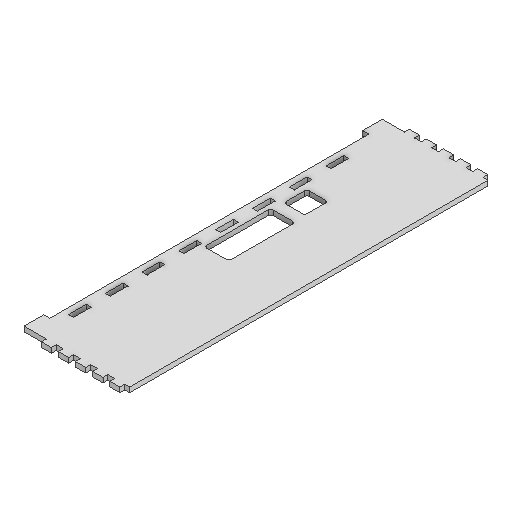
# Autodesk Inventor part: back
Saved by Autodesk Inventor 2025.2 (Build 292293000, 293)
## iProperties
Created: 2025-12-09
Part Number: back
Material: Generic
Document SubType Name: Modeling
Designer: hazem
Density: 1 g/cm^3
Appearance: Default
Author: hazem
Autodesk Inventor part; units mm, degrees
ref_plane "YZ Plane" through (0, 0, 0) normal (1, 0, 0) x (0, 1, 0)
ref_plane "XZ Plane" through (0, 0, 0) normal (0, 1, 0) x (-1, 0, 0)
ref_plane "XY Plane" through (0, 0, 0) normal (0, 0, 1) x (1, 0, 0)
sketch "Sketch1" plane through (0, 0, 0) normal (0, 1, 0) x (-1, 0, 0)
  line L0 (-71.6259, 7.6308) -> (8.4741, 7.6308)
  line L1 (8.4741, 7.6308) -> (8.4741, -292.3692)
  line L2 (8.4741, -292.3692) -> (-71.6259, -292.3692)
  line L3 (-71.6259, -292.3692) -> (-71.6259, 7.6308)
  point P0 (0, 0)
  constraints: 8 end point, 2 parallel, 1 horizontal, 1 perpendicular
extrude "Extrusion1" add sketch "Sketch1" along normal blind 4
sketch "Sketch2" plane through (0, 0, 0) normal (0, -1, 0) x (1, 0, 0)
  line L0 (-0.3741, 7.6308) -> (-18.4741, 7.6308) construction
  line L1 (-0.3741, 3.6308) -> (-0.3741, 7.6308) construction
  line L2 (7.6259, 7.6308) -> (7.6259, 3.6308) construction
  line L3 (13.6259, 3.6308) -> (7.6259, 3.6308) construction
  line L4 (13.6259, 3.6308) -> (13.6259, 7.6308) construction
  line L5 (21.6259, 7.6308) -> (21.6259, 3.6308) construction
  line L6 (27.6259, 3.6308) -> (21.6259, 3.6308) construction
  line L7 (27.6259, 3.6308) -> (27.6259, 7.6308) construction
  line L8 (35.6259, 7.6308) -> (35.6259, 3.6308) construction
  line L9 (41.6259, 3.6308) -> (35.6259, 3.6308) construction
  line L10 (41.6259, 3.6308) -> (41.6259, 7.6308) construction
  line L11 (49.6259, 7.6308) -> (49.6259, 3.6308) construction
  line L12 (55.6259, 3.6308) -> (49.6259, 3.6308) construction
  line L13 (55.6259, 3.6308) -> (55.6259, 7.6308) construction
  line L14 (63.6259, 7.6308) -> (63.6259, 3.6308) construction
  line L15 (67.6259, 3.6308) -> (63.6259, 3.6308) construction
  line L16 (67.6259, 7.6308) -> (67.6259, -292.3692) projected
  line L17 (71.6259, 7.6308) -> (71.6259, -292.3692) projected
  line L18 (67.6259, 7.6308) -> (67.6259, -292.3692) projected
  line L19 (71.6259, 7.6308) -> (71.6259, -292.3692) projected
  line L20 (67.6259, 7.6308) -> (67.6259, -292.3692) projected
  line L21 (71.6259, 7.6308) -> (71.6259, -292.3692) projected
  line L22 (67.6259, 7.6308) -> (67.6259, -292.3692) projected
  line L23 (71.6259, 7.6308) -> (71.6259, -292.3692) projected
  line L24 (67.6259, 7.6308) -> (67.6259, -292.3692) projected
  line L25 (71.6259, 7.6308) -> (71.6259, -292.3692) projected
  line L26 (67.6259, 7.6308) -> (67.6259, -292.3692) projected
  line L27 (71.6259, 7.6308) -> (71.6259, -292.3692) projected
  line L28 (67.6259, 7.6308) -> (67.6259, -292.3692) projected
  line L29 (71.6259, 7.6308) -> (71.6259, -292.3692) projected
  line L30 (67.6259, 7.6308) -> (67.6259, -292.3692) projected
  line L31 (71.6259, 7.6308) -> (71.6259, -292.3692) projected
  line L32 (67.6259, 7.6308) -> (67.6259, -292.3692) projected
  line L33 (71.6259, 7.6308) -> (71.6259, -292.3692) projected
  line L34 (67.6259, 7.6308) -> (67.6259, -292.3692) projected
  line L35 (71.6259, 7.6308) -> (71.6259, -292.3692) projected
  line L36 (13.5259, -288.3692) -> (7.5259, -288.3692) projected
  line L37 (55.5259, -292.3692) -> (55.5259, -288.3692) projected
  line L38 (55.5259, -288.3692) -> (49.5259, -288.3692) projected
  line L39 (49.5259, -288.3692) -> (49.5259, -292.3692) projected
  line L40 (41.5259, -288.3692) -> (35.5259, -288.3692) projected
  line L41 (41.5259, -292.3692) -> (41.5259, -288.3692) projected
  line L42 (35.5259, -288.3692) -> (35.5259, -292.3692) projected
  line L43 (27.5259, -288.3692) -> (21.5259, -288.3692) projected
  line L44 (27.5259, -292.3692) -> (27.5259, -288.3692) projected
  line L45 (21.5259, -288.3692) -> (21.5259, -292.3692) projected
  line L46 (13.5259, -288.3692) -> (7.5259, -288.3692) projected
  line L47 (13.5259, -292.3692) -> (13.5259, -288.3692) projected
  line L48 (7.5259, -288.3692) -> (7.5259, -292.3692) projected
  line L49 (-8.4741, -292.3692) -> (-8.4741, 7.6308) projected
  line L50 (-8.4741, -22.3692) -> (-8.4741, -37.3692) projected
  line L51 (-8.4741, -37.3692) -> (-4.4741, -37.3692) projected
  line L52 (-4.4741, -22.3692) -> (-4.4741, -37.3692) projected
  line L53 (-8.4741, -22.3692) -> (-4.4741, -22.3692) projected
  line L54 (-8.4741, -52.3692) -> (-8.4741, -67.3692) projected
  line L55 (-8.4741, -67.3692) -> (-4.4741, -67.3692) projected
  line L56 (-4.4741, -52.3692) -> (-4.4741, -67.3692) projected
  line L57 (-8.4741, -52.3692) -> (-4.4741, -52.3692) projected
  line L58 (-8.4741, -82.3692) -> (-8.4741, -97.3692) projected
  line L59 (-8.4741, -97.3692) -> (-4.4741, -97.3692) projected
  line L60 (-4.4741, -82.3692) -> (-4.4741, -97.3692) projected
  line L61 (-8.4741, -82.3692) -> (-4.4741, -82.3692) projected
  line L62 (-8.4741, -112.3692) -> (-8.4741, -127.3692) projected
  line L63 (-8.4741, -127.3692) -> (-4.4741, -127.3692) projected
  line L64 (-4.4741, -112.3692) -> (-4.4741, -127.3692) projected
  line L65 (-8.4741, -112.3692) -> (-4.4741, -112.3692) projected
  line L66 (-8.4741, -142.3692) -> (-8.4741, -157.3692) projected
  line L67 (-8.4741, -157.3692) -> (-4.4741, -157.3692) projected
  line L68 (-4.4741, -142.3692) -> (-4.4741, -157.3692) projected
  line L69 (-8.4741, -142.3692) -> (-4.4741, -142.3692) projected
  line L70 (-8.4741, -172.3692) -> (-8.4741, -187.3692) projected
  line L71 (-8.4741, -187.3692) -> (-4.4741, -187.3692) projected
  line L72 (-4.4741, -172.3692) -> (-4.4741, -187.3692) projected
  line L73 (-8.4741, -172.3692) -> (-4.4741, -172.3692) projected
  line L74 (-8.4741, -202.3692) -> (-8.4741, -217.3692) projected
  line L75 (-8.4741, -217.3692) -> (-4.4741, -217.3692) projected
  line L76 (-4.4741, -202.3692) -> (-4.4741, -217.3692) projected
  line L77 (-8.4741, -202.3692) -> (-4.4741, -202.3692) projected
  line L78 (-8.4741, -232.3692) -> (-8.4741, -247.3692) projected
  line L79 (-8.4741, -247.3692) -> (-4.4741, -247.3692) projected
  line L80 (-4.4741, -232.3692) -> (-4.4741, -247.3692) projected
  line L81 (-8.4741, -232.3692) -> (-4.4741, -232.3692) projected
  line L82 (71.6259, -37.1192) -> (67.6259, -37.1192)
  line L83 (67.6259, -22.6192) -> (71.6259, -22.6192)
  line L84 (67.6259, -52.6192) -> (71.6259, -52.6192)
  line L85 (71.6259, -67.1192) -> (67.6259, -67.1192)
  line L86 (67.6259, -82.6192) -> (71.6259, -82.6192)
  line L87 (71.6259, -97.1192) -> (67.6259, -97.1192)
  line L88 (67.6259, -112.6192) -> (71.6259, -112.6192)
  line L89 (71.6259, -127.1192) -> (67.6259, -127.1192)
  line L90 (67.6259, -142.6192) -> (71.6259, -142.6192)
  line L91 (71.6259, -157.1192) -> (67.6259, -157.1192)
  line L92 (67.6259, -172.6192) -> (71.6259, -172.6192)
  line L93 (71.6259, -187.1192) -> (67.6259, -187.1192)
  line L94 (67.6259, -202.6192) -> (71.6259, -202.6192)
  line L95 (71.6259, -217.1192) -> (67.6259, -217.1192)
  line L96 (67.6259, -232.6192) -> (71.6259, -232.6192)
  line L97 (71.6259, -247.1192) -> (67.6259, -247.1192)
  line L98 (67.6259, -262.6192) -> (71.6259, -262.6192)
  line L99 (71.6259, -277.1192) -> (67.6259, -277.1192)
  line L100 (-4.4741, -22.6192) -> (-8.4741, -22.6192)
  line L101 (-4.4741, -37.1192) -> (-8.4741, -37.1192)
  line L102 (-4.4741, -52.6192) -> (-8.4741, -52.6192)
  line L103 (-4.4741, -67.1192) -> (-8.4741, -67.1192)
  line L104 (-4.4741, -82.6192) -> (-8.4741, -82.6192)
  line L105 (-4.4741, -97.1192) -> (-8.4741, -97.1192)
  line L106 (-4.4741, -112.6192) -> (-8.4741, -112.6192)
  line L107 (-4.4741, -127.1192) -> (-8.4741, -127.1192)
  line L108 (-4.4741, -142.6192) -> (-8.4741, -142.6192)
  line L109 (-4.4741, -157.1192) -> (-8.4741, -157.1192)
  line L110 (-4.4741, -172.6192) -> (-8.4741, -172.6192)
  line L111 (-4.4741, -187.1192) -> (-8.4741, -187.1192)
  line L112 (-4.4741, -202.6192) -> (-8.4741, -202.6192)
  line L113 (-4.4741, -217.1192) -> (-8.4741, -217.1192)
  line L114 (-4.4741, -232.6192) -> (-8.4741, -232.6192)
  line L115 (-4.4741, -247.1192) -> (-8.4741, -247.1192)
  line L116 (7.8759, 7.6308) -> (7.8759, 3.6308)
  line L117 (13.3759, 3.6308) -> (13.3759, 7.6308)
  line L118 (21.8759, 7.6308) -> (21.8759, 3.6308)
  line L119 (27.3759, 3.6308) -> (27.3759, 7.6308)
  line L120 (35.8759, 7.6308) -> (35.8759, 3.6308)
  line L121 (41.3759, 3.6308) -> (41.3759, 7.6308)
  line L122 (49.8759, 7.6308) -> (49.8759, 3.6308)
  line L123 (55.3759, 3.6308) -> (55.3759, 7.6308)
  line L124 (7.7759, -292.3692) -> (7.7759, -288.3692)
  line L125 (13.2759, -288.3692) -> (13.2759, -292.3692)
  line L126 (21.7759, -292.3692) -> (21.7759, -288.3692)
  line L127 (27.2759, -288.3692) -> (27.2759, -292.3692)
  line L128 (35.7759, -292.3692) -> (35.7759, -288.3692)
  line L129 (41.2759, -288.3692) -> (41.2759, -292.3692)
  line L130 (49.7759, -292.3692) -> (49.7759, -288.3692)
  line L131 (55.2759, -288.3692) -> (55.2759, -292.3692)
  line L132 (13.6259, 3.6308) -> (7.6259, 3.6308) projected
  line L133 (27.6259, 3.6308) -> (21.6259, 3.6308) projected
  line L134 (41.6259, 3.6308) -> (35.6259, 3.6308) projected
  line L135 (55.6259, 3.6308) -> (49.6259, 3.6308) projected
  line L136 (71.6259, -292.3692) -> (-8.4741, -292.3692) projected
  line L137 (-0.3741, 3.6308) -> (-0.3741, 7.6308) projected
  line L138 (-8.4741, 7.6308) -> (71.6259, 7.6308) projected
  line L139 (71.6259, 7.6308) -> (71.6259, -292.3692) projected
  line L140 (63.6259, 7.6308) -> (63.6259, 3.6308) projected
  line L141 (67.6259, 3.6308) -> (63.6259, 3.6308) projected
  line L142 (-0.3741, 3.6308) -> (-18.4741, 3.6308) projected
  line L143 (-18.4741, 7.6308) -> (-18.4741, 3.6308) projected
  line L144 (-0.3741, 7.6308) -> (-18.4741, 7.6308) projected
  line L145 (-0.3741, 3.6308) -> (-0.3741, 7.6308) projected
  line L146 (-0.3741, 7.6308) -> (-18.4741, 7.6308) projected
  line L147 (-18.4741, 7.6308) -> (-18.4741, 3.6308) projected
  line L148 (-0.3741, 3.6308) -> (-18.4741, 3.6308) projected
  line L149 (-0.4741, -292.3692) -> (-0.4741, -288.3692) projected
  line L150 (-0.4741, -288.3692) -> (-18.4741, -288.3692) projected
  line L151 (-18.4741, -292.3692) -> (-18.4741, -288.3692) projected
  line L152 (-0.4741, -292.3692) -> (-18.4741, -292.3692) projected
  line L153 (15.6627, -189.1692) -> (2.2391, -189.1692)
  line L154 (0.3759, -191.0324) -> (0.3759, -206.206)
  line L155 (2.2391, -208.0692) -> (15.6627, -208.0692)
  line L156 (17.5259, -206.206) -> (17.5259, -191.0324)
  arc A0 (17.5259, -191.0324) -> (15.6627, -189.1692) centre (15.6627, -191.0324) ccw
  arc A1 (2.2391, -189.1692) -> (0.3759, -191.0324) centre (2.2391, -191.0324) ccw
  arc A2 (15.6627, -208.0692) -> (17.5259, -206.206) centre (15.6627, -206.206) ccw
  arc A3 (0.3759, -206.206) -> (2.2391, -208.0692) centre (2.2391, -206.206) ccw
  line L157 (16.9509, -125.8692) -> (0.9509, -125.8692)
  line L158 (-1.0491, -127.8692) -> (-1.0491, -177.8692)
  line L159 (0.9509, -179.8692) -> (16.9509, -179.8692)
  line L160 (18.9509, -177.8692) -> (18.9509, -127.8692)
  arc A4 (18.9509, -127.8692) -> (16.9509, -125.8692) centre (16.9509, -127.8692) ccw
  arc A5 (0.9509, -125.8692) -> (-1.0491, -127.8692) centre (0.9509, -127.8692) ccw
  arc A6 (16.9509, -179.8692) -> (18.9509, -177.8692) centre (16.9509, -177.8692) ccw
  arc A7 (-1.0491, -177.8692) -> (0.9509, -179.8692) centre (0.9509, -177.8692) ccw
  line L161 (67.6259, -292.3692) -> (71.6259, -292.3692) projected
  line L162 (67.6259, 7.6308) -> (71.6259, 7.6308) projected
  line L163 (67.6259, -292.3692) -> (71.6259, -292.3692) projected
  line L164 (67.6259, 7.6308) -> (71.6259, 7.6308) projected
  line L165 (67.6259, -292.3692) -> (71.6259, -292.3692) projected
  line L166 (67.6259, 7.6308) -> (71.6259, 7.6308) projected
  line L167 (67.6259, -292.3692) -> (71.6259, -292.3692) projected
  line L168 (67.6259, 7.6308) -> (71.6259, 7.6308) projected
  line L169 (67.6259, -292.3692) -> (71.6259, -292.3692) projected
  line L170 (67.6259, 7.6308) -> (71.6259, 7.6308) projected
  line L171 (67.6259, -292.3692) -> (71.6259, -292.3692) projected
  line L172 (67.6259, 7.6308) -> (71.6259, 7.6308) projected
  line L173 (67.6259, -292.3692) -> (71.6259, -292.3692) projected
  line L174 (67.6259, 7.6308) -> (71.6259, 7.6308) projected
  line L175 (67.6259, -292.3692) -> (71.6259, -292.3692) projected
  line L176 (67.6259, 7.6308) -> (71.6259, 7.6308) projected
  line L177 (67.6259, -292.3692) -> (71.6259, -292.3692) projected
  line L178 (67.6259, 7.6308) -> (71.6259, 7.6308) projected
  line L179 (67.6259, -292.3692) -> (71.6259, -292.3692) projected
  line L180 (67.6259, 7.6308) -> (71.6259, 7.6308) projected
  point P0 (0, 0)
  point P1 (71.6259, -7.3692)
  point P2 (71.6259, -37.3692)
  point P3 (71.6259, -22.3692)
  point P4 (71.6259, -67.3692)
  point P5 (71.6259, -52.3692)
  point P6 (71.6259, -97.3692)
  point P7 (71.6259, -82.3692)
  point P8 (71.6259, -127.3692)
  point P9 (71.6259, -112.3692)
  point P10 (71.6259, -157.3692)
  point P11 (71.6259, -142.3692)
  point P12 (71.6259, -187.3692)
  point P13 (71.6259, -172.3692)
  point P14 (71.6259, -217.3692)
  point P15 (71.6259, -202.3692)
  point P16 (71.6259, -247.3692)
  point P17 (71.6259, -232.3692)
  point P18 (71.6259, -277.3692)
  point P19 (71.6259, -262.3692)
  point P20 (67.6259, -97.1192)
  point P21 (71.6259, -97.1192)
  point P22 (71.6259, -82.6192)
  point P23 (67.6259, -82.6192)
  point P24 (67.6259, -127.1192)
  point P25 (71.6259, -127.1192)
  point P26 (71.6259, -112.6192)
  point P27 (67.6259, -112.6192)
  point P28 (67.6259, -157.1192)
  point P29 (71.6259, -157.1192)
  point P30 (71.6259, -142.6192)
  point P31 (67.6259, -142.6192)
  point P32 (67.6259, -187.1192)
  point P33 (71.6259, -187.1192)
  point P34 (71.6259, -172.6192)
  point P35 (67.6259, -172.6192)
  point P36 (67.6259, -217.1192)
  point P37 (71.6259, -217.1192)
  point P38 (71.6259, -202.6192)
  point P39 (67.6259, -202.6192)
  point P40 (67.6259, -247.1192)
  point P41 (71.6259, -247.1192)
  point P42 (71.6259, -232.6192)
  point P43 (67.6259, -232.6192)
  point P44 (67.6259, -277.1192)
  point P45 (71.6259, -277.1192)
  point P46 (71.6259, -262.6192)
  point P47 (67.6259, -262.6192)
  point P48 (-8.4741, -247.1192)
  point P49 (-4.4741, -247.1192)
  point P50 (-4.4741, -232.6192)
  point P51 (-8.4741, -232.6192)
  point P52 (-8.4741, -217.1192)
  point P53 (-4.4741, -217.1192)
  point P54 (-4.4741, -202.6192)
  point P55 (-8.4741, -202.6192)
  point P56 (-8.4741, -187.1192)
  point P57 (-4.4741, -187.1192)
  point P58 (-4.4741, -172.6192)
  point P59 (-8.4741, -172.6192)
  point P60 (-8.4741, -157.1192)
  point P61 (-4.4741, -157.1192)
  point P62 (-4.4741, -142.6192)
  point P63 (-8.4741, -142.6192)
  point P64 (-8.4741, -127.1192)
  point P65 (-4.4741, -127.1192)
  point P66 (-4.4741, -112.6192)
  point P67 (-8.4741, -112.6192)
  point P68 (-8.4741, -97.1192)
  point P69 (-4.4741, -97.1192)
  point P70 (-4.4741, -82.6192)
  point P71 (-8.4741, -82.6192)
  point P72 (-8.4741, -67.1192)
  point P73 (-4.4741, -67.1192)
  point P74 (-4.4741, -52.6192)
  point P75 (-8.4741, -52.6192)
  point P76 (-8.4741, -37.1192)
  point P77 (-8.4741, -22.6192)
  point P78 (67.6259, -67.1192)
  point P79 (71.6259, -67.1192)
  point P80 (71.6259, -52.6192)
  point P81 (67.6259, -52.6192)
  point P82 (8.9509, -189.1692)
  point P83 (8.9509, -179.8692)
  point P84 (67.6259, -292.3692)
  point P85 (67.6259, 3.6308)
  point P86 (67.6259, 7.6308)
  point P87 (71.6259, 3.6308)
  point P88 (67.6259, -288.3692)
  point P89 (71.6259, -288.3692)
  point P90 (-8.4741, 3.6308)
  point P91 (21.7759, -288.3692)
  point P92 (35.7759, -288.3692)
  point P93 (49.7759, -288.3692)
  point P94 (-8.4741, -288.3692)
  dimension "d7" = 30
  dimension "d15" = 30
  dimension "d20" = 0.25
  dimension "d23" = 14
  dimension "d28" = 0.25
  dimension "d31" = 14
  dimension "d49" = 2
  dimension "d50" = 50
  dimension "d51" = 20
  constraints: 118 end point, 16 point on circle, 16 tangent, 12 point on line, 8 centre point, 6 equal radius, 4 horizontal, 4 parallel, 4 perpendicular, 2 collinear, 2 midpoint, 2 vertical, 1 vertical alignment, 130 other
  measures "d7" distance of L83.start L84.start
  measures "d15" distance of L100.start L102.start
  measures "d20" distance between parallel lines of L2 L116
  measures "d23" distance of L116.start L118.start
  measures "d28" distance between parallel lines of L48 L124
  measures "d31" distance of L124.start L126.start
  measures "d49" radius of A4
  measures "d50" distance of L160.start L160.end
  measures "d51" distance between parallel lines of L158 L160
extrude "Extrusion2" cut sketch "Sketch2" against normal through all contours L138 L17 L83 L16 | L16 L141 L140 L138 | L83 L17 L82 L16 | L123 L135 L122 L138 | L82 L17 L84 L16 | L84 L17 L85 L16 | L121 L134 L120 L138 | L85 L17 L86 L16 | L86 L17 L87 L16 | L119 L133 L118 L138 | L87 L17 L88 L16 | L88 L17 L89 L16 | L117 L132 L116 L138 | L89 L17 L90 L16 | L90 L17 L91 L16 | L137 L142 L49 L138 | L91 L17 L92 L16 | L92 L17 L93 L16 | L93 L17 L94 L16 | L94 L17 L95 L16 | L100 L52 L101 L49 | L95 L17 L96 L16 | L96 L17 L97 L16 | L97 L17 L98 L16 | L98 L17 L99 L16 | L102 L56 L103 L49 | L99 L17 L136 L16 | L136 L130 L38 L131 | L104 L60 L105 L49 | L136 L128 L40 L129 | L106 L64 L107 L49 | L136 L126 L43 L127 | L108 L68 L109 L49 | L136 L124 L36 L125 | L110 L72 L111 L49 | L136 L49 L150 L149 | L112 L76 L113 L49 | L49 L114 L80 L115 | A0 L156 A2 L155 A3 L154 A1 L153 | A4 L160 A6 L159 A7 L158 A5 L157
sketch "Sketch3" plane through (0, 0, 0) normal (0, -1, 0) x (1, 0, 0)
  line L0 (-8.4741, 7.6308) -> (7.8759, 7.6308) projected
  line L1 (7.7759, -292.3692) -> (-8.4741, -292.3692) projected
  line L2 (-8.4741, -22.6192) -> (-8.4741, 3.6308) projected
  line L3 (-8.4741, 3.6308) -> (-18.4741, 3.6308)
  line L4 (-18.4741, 3.6308) -> (-18.4741, -12.3692)
  line L5 (-18.4741, -12.3692) -> (-8.4741, -12.3692)
  line L6 (-8.4741, -12.3692) -> (-8.4741, 3.6308)
  line L7 (-8.4741, -292.3692) -> (-8.4741, -247.1192) projected
  line L8 (-8.4741, -288.3692) -> (-18.4741, -288.3692)
  line L9 (-18.4741, -288.3692) -> (-18.4741, -272.3692)
  line L10 (-18.4741, -272.3692) -> (-8.4741, -272.3692)
  line L11 (-8.4741, -272.3692) -> (-8.4741, -288.3692)
  line L12 (-8.4741, -12.3692) -> (-8.4741, -272.3692)
  line L13 (49.8759, 3.6308) -> (49.8759, 7.6308) projected
  line L14 (41.3759, 7.6308) -> (49.8759, 7.6308) projected
  line L15 (41.3759, 7.6308) -> (41.3759, 3.6308) projected
  line L16 (41.3759, 3.6308) -> (35.8759, 3.6308) projected
  line L17 (35.8759, 3.6308) -> (35.8759, 7.6308) projected
  line L18 (27.3759, 7.6308) -> (35.8759, 7.6308) projected
  line L19 (27.3759, 7.6308) -> (27.3759, 3.6308) projected
  line L20 (27.3759, 3.6308) -> (21.8759, 3.6308) projected
  line L21 (21.8759, 3.6308) -> (21.8759, 7.6308) projected
  line L22 (13.3759, 7.6308) -> (21.8759, 7.6308) projected
  line L23 (13.3759, 7.6308) -> (13.3759, 3.6308) projected
  line L24 (13.3759, 3.6308) -> (7.8759, 3.6308) projected
  line L25 (7.8759, 3.6308) -> (7.8759, 7.6308) projected
  line L26 (-0.3741, 7.6308) -> (7.8759, 7.6308) projected
  line L27 (-0.3741, 7.6308) -> (-0.3741, 3.6308) projected
  line L28 (-0.3741, 3.6308) -> (-8.4741, 3.6308) projected
  line L29 (-8.4741, -22.6192) -> (-8.4741, 3.6308) projected
  line L30 (-4.4741, -22.6192) -> (-4.4741, -37.1192) projected
  line L31 (-8.4741, -52.6192) -> (-8.4741, -37.1192) projected
  line L32 (-4.4741, -52.6192) -> (-4.4741, -67.1192) projected
  line L33 (-8.4741, -82.6192) -> (-8.4741, -67.1192) projected
  line L34 (-4.4741, -82.6192) -> (-4.4741, -97.1192) projected
  line L35 (-8.4741, -112.6192) -> (-8.4741, -97.1192) projected
  line L36 (-4.4741, -112.6192) -> (-4.4741, -127.1192) projected
  line L37 (-8.4741, -142.6192) -> (-8.4741, -127.1192) projected
  line L38 (-4.4741, -142.6192) -> (-4.4741, -157.1192) projected
  line L39 (-8.4741, -172.6192) -> (-8.4741, -157.1192) projected
  line L40 (-4.4741, -172.6192) -> (-4.4741, -187.1192) projected
  line L41 (-8.4741, -202.6192) -> (-8.4741, -187.1192) projected
  line L42 (-4.4741, -202.6192) -> (-4.4741, -217.1192) projected
  line L43 (-8.4741, -232.6192) -> (-8.4741, -217.1192) projected
  line L44 (-4.4741, -232.6192) -> (-4.4741, -247.1192) projected
  line L45 (-8.4741, -288.3692) -> (-8.4741, -247.1192) projected
  line L46 (7.7759, -292.3692) -> (-0.4741, -292.3692) projected
  line L47 (7.7759, -288.3692) -> (13.2759, -288.3692) projected
  line L48 (21.7759, -292.3692) -> (13.2759, -292.3692) projected
  line L49 (67.6259, -292.3692) -> (67.6259, 3.6308) projected
  line L50 (55.3759, 7.6308) -> (63.6259, 7.6308) projected
  line L51 (55.3759, 7.6308) -> (55.3759, 3.6308) projected
  line L52 (55.3759, 3.6308) -> (49.8759, 3.6308) projected
  line L53 (-13.4741, -12.3692) -> (-13.4741, -272.3692)
  line L54 (67.6259, 3.6308) -> (63.6259, 3.6308) projected
  line L55 (63.6259, 3.6308) -> (63.6259, 7.6308) projected
  line L56 (-8.4741, -22.6192) -> (-4.4741, -22.6192) projected
  line L57 (-4.4741, -37.1192) -> (-8.4741, -37.1192) projected
  line L58 (-8.4741, -52.6192) -> (-4.4741, -52.6192) projected
  line L59 (-4.4741, -67.1192) -> (-8.4741, -67.1192) projected
  line L60 (-8.4741, -82.6192) -> (-4.4741, -82.6192) projected
  line L61 (-4.4741, -97.1192) -> (-8.4741, -97.1192) projected
  line L62 (-8.4741, -112.6192) -> (-4.4741, -112.6192) projected
  line L63 (-4.4741, -127.1192) -> (-8.4741, -127.1192) projected
  line L64 (-8.4741, -142.6192) -> (-4.4741, -142.6192) projected
  line L65 (-4.4741, -157.1192) -> (-8.4741, -157.1192) projected
  line L66 (-8.4741, -172.6192) -> (-4.4741, -172.6192) projected
  line L67 (-4.4741, -187.1192) -> (-8.4741, -187.1192) projected
  line L68 (-8.4741, -202.6192) -> (-4.4741, -202.6192) projected
  line L69 (-4.4741, -217.1192) -> (-8.4741, -217.1192) projected
  line L70 (-8.4741, -232.6192) -> (-4.4741, -232.6192) projected
  line L71 (-4.4741, -247.1192) -> (-8.4741, -247.1192) projected
  line L72 (7.7759, -292.3692) -> (7.7759, -288.3692) projected
  line L73 (13.2759, -288.3692) -> (13.2759, -292.3692) projected
  line L74 (27.2759, -288.3692) -> (27.2759, -292.3692) projected
  line L75 (35.7759, -292.3692) -> (27.2759, -292.3692) projected
  line L76 (35.7759, -292.3692) -> (35.7759, -288.3692) projected
  line L77 (35.7759, -288.3692) -> (41.2759, -288.3692) projected
  line L78 (41.2759, -288.3692) -> (41.2759, -292.3692) projected
  line L79 (49.7759, -292.3692) -> (41.2759, -292.3692) projected
  line L80 (49.7759, -292.3692) -> (49.7759, -288.3692) projected
  line L81 (49.7759, -288.3692) -> (55.2759, -288.3692) projected
  line L82 (55.2759, -288.3692) -> (55.2759, -292.3692) projected
  line L83 (67.6259, -292.3692) -> (55.2759, -292.3692) projected
  line L84 (21.7759, -292.3692) -> (21.7759, -288.3692) projected
  line L85 (21.7759, -288.3692) -> (27.2759, -288.3692) projected
  line L86 (-8.4741, -288.3692) -> (-0.4741, -288.3692) projected
  line L87 (-0.4741, -288.3692) -> (-0.4741, -292.3692) projected
  point P0 (0, 0)
  point P1 (7.5259, -292.3692)
  point P2 (-8.4741, -22.3692)
  point P3 (-8.4741, -247.3692)
  point P4 (-8.4741, -247.1192)
  point P5 (-8.4741, -22.6192)
  dimension "d44" = 20
  dimension "d45" = 10
  dimension "d46" = 5
  constraints: 20 end point, 4 parallel, 3 perpendicular, 2 equal length, 2 horizontal, 2 midpoint, 1 vertical
  measures "d44" distance between parallel lines of L0 L5
  measures "d45" distance of L2.end L3.end
  measures "d46" distance between parallel lines of L53 L12
extrude "Extrusion3" add sketch "Sketch3" against normal up to surface (4 mm away) contours L2 L5 L4 L3 | L2 L12 L7 L10 L53 L5 | L10 L7 L8 L9
sketch "Sketch4" plane through (0, 4, 0) normal (0, 1, 0) x (1, 0, 0)
  line L0 (-8.4741, 67.1192) -> (-4.4741, 67.1192) projected
  line L1 (-4.4741, 67.1192) -> (-4.4741, 52.6192) projected
  line L2 (-4.4741, 52.6192) -> (-8.4741, 52.6192) projected
  line L3 (-8.4741, 67.1192) -> (-8.4741, 52.6192) projected
  line L4 (-8.4741, 247.1192) -> (-4.4741, 247.1192) projected
  line L5 (-4.4741, 247.1192) -> (-4.4741, 232.6192) projected
  line L6 (-4.4741, 232.6192) -> (-8.4741, 232.6192) projected
  line L7 (-8.4741, 247.1192) -> (-8.4741, 232.6192) projected
  line L8 (-8.4741, 97.1192) -> (-8.4741, 82.6192) projected
  line L9 (-8.4741, 97.1192) -> (-4.4741, 97.1192) projected
  line L10 (-4.4741, 97.1192) -> (-4.4741, 82.6192) projected
  line L11 (-4.4741, 82.6192) -> (-8.4741, 82.6192) projected
  line L12 (-18.4741, 288.3692) -> (-0.4741, 288.3692) projected
  line L13 (-18.4741, 272.3692) -> (-18.4741, 288.3692) projected
  line L14 (-13.4741, 272.3692) -> (-18.4741, 272.3692) projected
  line L15 (-13.4741, 12.3692) -> (-13.4741, 272.3692) projected
  line L16 (-18.4741, 12.3692) -> (-13.4741, 12.3692) projected
  line L17 (-18.4741, -3.6308) -> (-18.4741, 12.3692) projected
  line L18 (-18.4741, -3.6308) -> (-0.3741, -3.6308) projected
  line L19 (-0.3741, -3.6308) -> (-0.3741, -7.6308) projected
  line L20 (-0.3741, -7.6308) -> (7.8759, -7.6308) projected
  line L21 (7.8759, -7.6308) -> (7.8759, -3.6308) projected
  line L22 (7.8759, -3.6308) -> (13.3759, -3.6308) projected
  line L23 (13.3759, -3.6308) -> (13.3759, -7.6308) projected
  line L24 (13.3759, -7.6308) -> (21.8759, -7.6308) projected
  line L25 (21.8759, -7.6308) -> (21.8759, -3.6308) projected
  line L26 (21.8759, -3.6308) -> (27.3759, -3.6308) projected
  line L27 (27.3759, -3.6308) -> (27.3759, -7.6308) projected
  line L28 (27.3759, -7.6308) -> (35.8759, -7.6308) projected
  line L29 (35.8759, -7.6308) -> (35.8759, -3.6308) projected
  line L30 (35.8759, -3.6308) -> (41.3759, -3.6308) projected
  line L31 (41.3759, -3.6308) -> (41.3759, -7.6308) projected
  line L32 (41.3759, -7.6308) -> (49.8759, -7.6308) projected
  line L33 (49.8759, -7.6308) -> (49.8759, -3.6308) projected
  line L34 (49.8759, -3.6308) -> (55.3759, -3.6308) projected
  line L35 (55.3759, -3.6308) -> (55.3759, -7.6308) projected
  line L36 (55.3759, -7.6308) -> (63.6259, -7.6308) projected
  line L37 (63.6259, -7.6308) -> (63.6259, -3.6308) projected
  line L38 (63.6259, -3.6308) -> (67.6259, -3.6308) projected
  line L39 (67.6259, -3.6308) -> (67.6259, 292.3692) projected
  line L40 (67.6259, 292.3692) -> (55.2759, 292.3692) projected
  line L41 (55.2759, 292.3692) -> (55.2759, 288.3692) projected
  line L42 (55.2759, 288.3692) -> (49.7759, 288.3692) projected
  line L43 (49.7759, 288.3692) -> (49.7759, 292.3692) projected
  line L44 (49.7759, 292.3692) -> (41.2759, 292.3692) projected
  line L45 (41.2759, 292.3692) -> (41.2759, 288.3692) projected
  line L46 (41.2759, 288.3692) -> (35.7759, 288.3692) projected
  line L47 (35.7759, 288.3692) -> (35.7759, 292.3692) projected
  line L48 (35.7759, 292.3692) -> (27.2759, 292.3692) projected
  line L49 (27.2759, 292.3692) -> (27.2759, 288.3692) projected
  line L50 (27.2759, 288.3692) -> (21.7759, 288.3692) projected
  line L51 (21.7759, 288.3692) -> (21.7759, 292.3692) projected
  line L52 (21.7759, 292.3692) -> (13.2759, 292.3692) projected
  line L53 (13.2759, 292.3692) -> (13.2759, 288.3692) projected
  line L54 (13.2759, 288.3692) -> (7.7759, 288.3692) projected
  line L55 (7.7759, 288.3692) -> (7.7759, 292.3692) projected
  line L56 (7.7759, 292.3692) -> (-0.4741, 292.3692) projected
  line L57 (-0.4741, 292.3692) -> (-0.4741, 288.3692) projected
  line L58 (-8.4741, 37.1192) -> (-8.4741, 22.6192) projected
  line L59 (-8.4741, 37.1192) -> (-4.4741, 37.1192) projected
  line L60 (-4.4741, 37.1192) -> (-4.4741, 22.6192) projected
  line L61 (-4.4741, 22.6192) -> (-8.4741, 22.6192) projected
  line L62 (-8.4741, 127.1192) -> (-8.4741, 112.6192) projected
  line L63 (-8.4741, 127.1192) -> (-4.4741, 127.1192) projected
  line L64 (-4.4741, 127.1192) -> (-4.4741, 112.6192) projected
  line L65 (-4.4741, 112.6192) -> (-8.4741, 112.6192) projected
  line L66 (-8.4741, 157.1192) -> (-8.4741, 142.6192) projected
  line L67 (-8.4741, 157.1192) -> (-4.4741, 157.1192) projected
  line L68 (-4.4741, 157.1192) -> (-4.4741, 142.6192) projected
  line L69 (-4.4741, 142.6192) -> (-8.4741, 142.6192) projected
  line L70 (-8.4741, 187.1192) -> (-8.4741, 172.6192) projected
  line L71 (-8.4741, 187.1192) -> (-4.4741, 187.1192) projected
  line L72 (-4.4741, 187.1192) -> (-4.4741, 172.6192) projected
  line L73 (-4.4741, 172.6192) -> (-8.4741, 172.6192) projected
  line L74 (0.3759, 191.0324) -> (0.3759, 206.206) projected
  arc A0 (2.2391, 208.0692) -> (0.3759, 206.206) centre (2.2391, 206.206) ccw projected
  line L75 (2.2391, 208.0692) -> (15.6627, 208.0692) projected
  arc A1 (17.5259, 206.206) -> (15.6627, 208.0692) centre (15.6627, 206.206) ccw projected
  line L76 (17.5259, 206.206) -> (17.5259, 191.0324) projected
  arc A2 (15.6627, 189.1692) -> (17.5259, 191.0324) centre (15.6627, 191.0324) ccw projected
  line L77 (15.6627, 189.1692) -> (2.2391, 189.1692) projected
  arc A3 (0.3759, 191.0324) -> (2.2391, 189.1692) centre (2.2391, 191.0324) ccw projected
  line L78 (-1.0491, 127.8692) -> (-1.0491, 177.8692) projected
  arc A4 (0.9509, 179.8692) -> (-1.0491, 177.8692) centre (0.9509, 177.8692) ccw projected
  line L79 (0.9509, 179.8692) -> (16.9509, 179.8692) projected
  arc A5 (18.9509, 177.8692) -> (16.9509, 179.8692) centre (16.9509, 177.8692) ccw projected
  line L80 (18.9509, 177.8692) -> (18.9509, 127.8692) projected
  arc A6 (16.9509, 125.8692) -> (18.9509, 127.8692) centre (16.9509, 127.8692) ccw projected
  line L81 (16.9509, 125.8692) -> (0.9509, 125.8692) projected
  arc A7 (-1.0491, 127.8692) -> (0.9509, 125.8692) centre (0.9509, 127.8692) ccw projected
  line L82 (-8.4741, 217.1192) -> (-8.4741, 202.6192) projected
  line L83 (-8.4741, 217.1192) -> (-4.4741, 217.1192) projected
  line L84 (-4.4741, 217.1192) -> (-4.4741, 202.6192) projected
  line L85 (-4.4741, 202.6192) -> (-8.4741, 202.6192) projected
  line L86 (63.6259, 292.3692) -> (63.6259, 288.3692)
  line L87 (63.6259, 288.3692) -> (67.6259, 288.3692)
  line L88 (67.6259, -3.6308) -> (67.6259, 292.3692) projected
  point P0 (0, 0)
  dimension "d52" = 4
  dimension "d53" = 4
  constraints: 4 end point, 2 point on line, 1 perpendicular, 1 vertical
  measures "d52" distance of L86.start L86.end
  measures "d53" distance of L86.end L87.end
extrude "Extrusion4" cut sketch "Sketch4" against normal through all contours L40 L39 L87 L86
body "Solid1"
